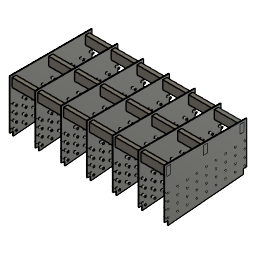
_Shelf Assembly for Animation.40ab5e80-e004-40ce-8bc8-a0c1a8f30ea9 (Autodesk Fusion 360 design; units mm, degrees)
Autodesk Fusion 360 part; units mm, degrees
sketch "Sketch1" plane through (0, 0, 0) normal (0, 0, 1) x (1, 0, 0)
  line L0 (0, 0) -> (6.35, 0)
  line L1 (6.35, 0) -> (6.35, 958.998)
  line L2 (6.35, 1060.598) -> (0, 1060.598)
  line L3 (0, 1060.598) -> (0, 0)
  line L4 (292.7, 0) -> (292.7, 958.998)
  line L5 (286.35, 0) -> (292.7, 0)
  line L6 (286.35, 958.998) -> (286.35, 0)
  line L7 (292.7, 1060.598) -> (286.35, 1060.598)
  line L8 (579.05, 0) -> (579.05, 958.998)
  line L9 (572.7, 0) -> (579.05, 0)
  line L10 (572.7, 958.998) -> (572.7, 0)
  line L11 (579.05, 1060.598) -> (572.7, 1060.598)
  line L12 (865.4, 0) -> (865.4, 958.998)
  line L13 (859.05, 0) -> (865.4, 0)
  line L14 (859.05, 958.998) -> (859.05, 0)
  line L15 (865.4, 1060.598) -> (859.05, 1060.598)
  line L16 (1151.75, 0) -> (1151.75, 958.998)
  line L17 (1145.4, 0) -> (1151.75, 0)
  line L18 (1145.4, 958.998) -> (1145.4, 0)
  line L19 (1151.75, 1060.598) -> (1145.4, 1060.598)
  line L20 (1438.1, 0) -> (1438.1, 958.998)
  line L21 (1431.75, 0) -> (1438.1, 0)
  line L22 (1431.75, 958.998) -> (1431.75, 0)
  line L23 (1438.1, 1060.598) -> (1431.75, 1060.598)
  line L24 (1724.45, 0) -> (1724.45, 1060.598)
  line L25 (1718.1, 0) -> (1724.45, 0)
  line L26 (1718.1, 958.998) -> (1718.1, 0)
  line L27 (1724.45, 1060.598) -> (1718.1, 1060.598)
  line L28 (0, 1060.598) -> (1724.45, 1060.598)
  line L29 (1724.45, 1060.598) -> (1724.45, 958.998)
  line L30 (0, 958.998) -> (0, 1060.598)
  line L31 (286.35, 958.998) -> (6.35, 958.998)
  line L32 (572.7, 958.998) -> (292.7, 958.998)
  line L33 (859.05, 958.998) -> (579.05, 958.998)
  line L34 (1145.4, 958.998) -> (865.4, 958.998)
  line L35 (1718.1, 958.998) -> (1438.1, 958.998)
  line L36 (1431.75, 958.998) -> (1151.75, 958.998)
  point P0 (286.35, 0)
  point P1 (572.7, 0)
  point P2 (859.05, 0)
  point P3 (1145.4, 0)
  point P4 (1431.75, 0)
  point P5 (1718.1, 0)
  dimension "d1" = 6.35
  dimension "d2" = 1060.598
  dimension "d7" = 101.6
  constraint horizontal L0
  constraint vertical L1
  constraint horizontal L2
  constraint vertical L3
  constraint coincident L0.start L3.end
  constraint horizontal L28
  constraint vertical L29
  constraint horizontal L35
  constraint vertical L30
  constraint coincident L24 L29.end
  constraint coincident L6.start L35
  constraint coincident L10.start L35
  constraint coincident L14.start L35
  constraint coincident L18.start L35
  constraint coincident L22.start L35
  constraint collinear L31 L35
  constraint collinear L32 L35
  constraint collinear L33 L35
  constraint collinear L34 L35
  constraint collinear L35 L36
  measures "d1" distance of L0.start L0.end
  measures "d2" distance of L0.start L2.end
  measures "d7" distance of L2.end L30.start
sketch "Sketch3" plane through (0, 0, 0) normal (1, 0, 0) x (0, 0, -1)
  circle A0 centre (-408.3427, 236.1947) radius 5.3675
  circle A1 centre (-195.157, 334.846) radius 5.3675
  line L0 (-380.15, 576.0244) -> (-380.15, 480.7744)
  line L1 (-380.15, 480.7744) -> (-424.6, 480.7744)
  circle A2 centre (-301.7498, 325.5203) radius 5.3675
  line L2 (-411.9, 3.3333) -> (426.3, 76.6663)
  line L3 (-424.6, 576.024) -> (-380.15, 576.0244)
  circle A3 centre (-301.7498, 245.5203) radius 5.3675
  line L4 (464.4, 600.8) -> (-450, 600.8)
  circle A4 centre (-435, 328.3) radius 2.25
  circle A5 centre (-195.157, 254.846) radius 5.3675
  line L5 (-424.6, 480.7744) -> (-424.6, 576.024)
  circle A6 centre (-408.3427, 316.1947) radius 5.3675
  circle A7 centre (-435, 248.3) radius 2.25
  circle A8 centre (124.6215, 282.823) radius 5.3675
  circle A9 centre (337.8072, 381.4743) radius 5.3675
  circle A10 centre (-88.5642, 344.1717) radius 5.3675
  line L6 (-450, 50.8) -> (-411.9, 50.8)
  circle A11 centre (18.0287, 353.4973) radius 5.3675
  line L7 (390.4, 576.024) -> (434.85, 576.0244)
  circle A12 centre (-408.3427, 76.1947) radius 5.3675
  circle A13 centre (-435, 88.3) radius 2.25
  line L8 (426.3, 76.6663) -> (426.3, 130.7996)
  circle A14 centre (337.8072, 141.4743) radius 5.3675
  circle A15 centre (18.0287, 193.4973) radius 5.3675
  circle A16 centre (231.2143, 132.1487) radius 5.3675
  circle A17 centre (444.4, 310.8) radius 5.3675
  circle A18 centre (124.6215, 362.823) radius 5.3675
  line L9 (390.4, 480.7744) -> (390.4, 576.024)
  circle A19 centre (18.0287, 273.4973) radius 5.3675
  line L10 (434.85, 480.7744) -> (390.4, 480.7744)
  circle A20 centre (-195.157, 174.846) radius 5.3675
  circle A21 centre (-301.7498, 85.5203) radius 5.3675
  line L11 (27.35, 480.7744) -> (-17.1, 480.7744)
  line L12 (426.3, 130.7996) -> (464.4, 130.7996)
  line L13 (-17.1, 576.024) -> (27.35, 576.0244)
  circle A22 centre (444.4, 150.8) radius 5.3675
  circle A23 centre (-301.7498, 165.5203) radius 5.3675
  line L14 (-411.9, 50.8) -> (-411.9, 3.3333)
  circle A24 centre (444.4, 230.8) radius 5.3675
  circle A25 centre (-408.3427, 156.1947) radius 5.3675
  circle A26 centre (-195.157, 94.846) radius 5.3675
  circle A27 centre (-435, 168.3) radius 2.25
  line L15 (-17.1, 480.7744) -> (-17.1, 576.024)
  line L16 (-450, 600.8) -> (-450, 50.8)
  circle A28 centre (18.0287, 113.4973) radius 5.3675
  circle A29 centre (231.2143, 372.1487) radius 5.3675
  circle A30 centre (-88.5642, 184.1717) radius 5.3675
  circle A31 centre (444.4, 390.8) radius 5.3675
  circle A32 centre (337.8072, 301.4743) radius 5.3675
  circle A33 centre (337.8072, 221.4743) radius 5.3675
  line L17 (464.4, 130.7996) -> (464.4, 600.8)
  circle A34 centre (231.2143, 212.1487) radius 5.3675
  line L18 (434.85, 576.0244) -> (434.85, 480.7744)
  circle A35 centre (-88.5642, 104.1717) radius 5.3675
  circle A36 centre (124.6215, 122.823) radius 5.3675
  circle A37 centre (124.6215, 202.823) radius 5.3675
  line L19 (27.35, 576.0244) -> (27.35, 480.7744)
  circle A38 centre (-88.5642, 264.1717) radius 5.3675
  circle A39 centre (231.2143, 292.1487) radius 5.3675
  point P0 (-100, 0)
extrude "Extrude2" add sketch "Sketch3" along normal blind 6.35 makes body 1
pattern_linear "R-Pattern1" count 7 spacing 286.35 along (1, 0, 0) of bodies 1 makes body 2 at (286.35, 509.8549, -216.3214) makes body 3 at (572.7, 509.8549, -216.3214) makes body 4 at (859.05, 509.8549, -216.3214) makes body 5 at (1145.4, 509.8549, -216.3214) makes body 6 at (1431.75, 509.8549, -216.3214) makes body 7 at (1718.1, 509.8549, -216.3214)
sketch "Sketch4" plane through (0, 0, 0) normal (-1, 0, 0) x (0, 0, 1)
  circle A0 centre (-124.6215, 202.823) radius 5.3675
  circle A1 centre (408.3427, 156.1947) radius 5.3675
  circle A2 centre (-444.4, 310.8) radius 5.3675
  circle A3 centre (-337.8072, 221.4743) radius 5.3675
  circle A4 centre (-231.2143, 132.1487) radius 5.3675
  circle A5 centre (435, 168.3) radius 2.25
  circle A6 centre (-231.2143, 292.1487) radius 5.3675
  circle A7 centre (-124.6215, 122.823) radius 5.3675
  circle A8 centre (-444.4, 150.8) radius 5.3675
  line L0 (-434.85, 576.0244) -> (-390.4, 576.024)
  line L1 (-390.4, 576.024) -> (-390.4, 480.7744)
  line L2 (-390.4, 480.7744) -> (-434.85, 480.7744)
  line L3 (-434.85, 480.7744) -> (-434.85, 576.0244)
  circle A9 centre (-337.8072, 301.4743) radius 5.3675
  circle A10 centre (195.157, 94.846) radius 5.3675
  circle A11 centre (301.7498, 245.5203) radius 5.3675
  circle A12 centre (301.7498, 85.5203) radius 5.3675
  circle A13 centre (-18.0287, 113.4973) radius 5.3675
  circle A14 centre (301.7498, 165.5203) radius 5.3675
  circle A15 centre (-444.4, 230.8) radius 5.3675
  circle A16 centre (88.5642, 104.1717) radius 5.3675
  circle A17 centre (-231.2143, 212.1487) radius 5.3675
  circle A18 centre (88.5642, 184.1717) radius 5.3675
  circle A19 centre (88.5642, 264.1717) radius 5.3675
  circle A20 centre (-337.8072, 141.4743) radius 5.3675
  circle A21 centre (-231.2143, 372.1487) radius 5.3675
  line L4 (424.6, 480.7744) -> (380.15, 480.7744)
  line L5 (380.15, 480.7744) -> (380.15, 576.0244)
  line L6 (380.15, 576.0244) -> (424.6, 576.024)
  line L7 (424.6, 576.024) -> (424.6, 480.7744)
  circle A22 centre (-124.6215, 362.823) radius 5.3675
  circle A23 centre (195.157, 334.846) radius 5.3675
  circle A24 centre (435, 88.3) radius 2.25
  circle A25 centre (408.3427, 236.1947) radius 5.3675
  circle A26 centre (435, 328.3) radius 2.25
  circle A27 centre (195.157, 254.846) radius 5.3675
  circle A28 centre (195.157, 174.846) radius 5.3675
  circle A29 centre (-444.4, 390.8) radius 5.3675
  circle A30 centre (-18.0287, 193.4973) radius 5.3675
  line L8 (-27.35, 576.0244) -> (17.1, 576.024)
  line L9 (17.1, 576.024) -> (17.1, 480.7744)
  line L10 (17.1, 480.7744) -> (-27.35, 480.7744)
  line L11 (-27.35, 480.7744) -> (-27.35, 576.0244)
  circle A31 centre (-18.0287, 273.4973) radius 5.3675
  circle A32 centre (408.3427, 76.1947) radius 5.3675
  circle A33 centre (435, 248.3) radius 2.25
  circle A34 centre (-337.8072, 381.4743) radius 5.3675
  circle A35 centre (-124.6215, 282.823) radius 5.3675
  circle A36 centre (301.7498, 325.5203) radius 5.3675
  circle A37 centre (88.5642, 344.1717) radius 5.3675
  circle A38 centre (-18.0287, 353.4973) radius 5.3675
  circle A39 centre (408.3427, 316.1947) radius 5.3675
  line L12 (-464.4, 600.8) -> (-464.4, 130.7996)
  line L13 (-464.4, 130.7996) -> (-426.3, 130.7996)
  line L14 (-426.3, 130.7996) -> (-426.3, 76.6663)
  line L15 (-426.3, 76.6663) -> (411.9, 3.3333)
  line L16 (411.9, 3.3333) -> (411.9, 50.8)
  line L17 (411.9, 50.8) -> (450, 50.8)
  line L18 (450, 50.8) -> (450, 600.8)
  line L19 (450, 600.8) -> (-464.4, 600.8)
extrude "Extrude3" add sketch "Sketch4" against normal up to surface (1724.45 mm away) contours L0 L1 L2 L3 | L4 L5 L6 L7 | L8 L9 L10 L11 bodies 1 2 3 4 5 6 7
sketch "Sketch5" plane through (0, 0, 0) normal (-1, 0, 0) x (0, 0, 1)
  circle A0 centre (-124.6215, 202.823) radius 5.3675
  circle A1 centre (408.3427, 156.1947) radius 5.3675
  circle A2 centre (-444.4, 310.8) radius 5.3675
  circle A3 centre (-337.8072, 221.4743) radius 5.3675
  circle A4 centre (-231.2143, 132.1487) radius 5.3675
  circle A5 centre (435, 168.3) radius 2.25
  circle A6 centre (-231.2143, 292.1487) radius 5.3675
  circle A7 centre (-124.6215, 122.823) radius 5.3675
  circle A8 centre (-444.4, 150.8) radius 5.3675
  circle A9 centre (-337.8072, 301.4743) radius 5.3675
  circle A10 centre (195.157, 94.846) radius 5.3675
  circle A11 centre (301.7498, 245.5203) radius 5.3675
  circle A12 centre (301.7498, 85.5203) radius 5.3675
  circle A13 centre (-18.0287, 113.4973) radius 5.3675
  circle A14 centre (301.7498, 165.5203) radius 5.3675
  circle A15 centre (-444.4, 230.8) radius 5.3675
  circle A16 centre (88.5642, 104.1717) radius 5.3675
  circle A17 centre (-231.2143, 212.1487) radius 5.3675
  circle A18 centre (88.5642, 184.1717) radius 5.3675
  circle A19 centre (88.5642, 264.1717) radius 5.3675
  circle A20 centre (-337.8072, 141.4743) radius 5.3675
  circle A21 centre (-231.2143, 372.1487) radius 5.3675
  circle A22 centre (-124.6215, 362.823) radius 5.3675
  circle A23 centre (195.157, 334.846) radius 5.3675
  circle A24 centre (435, 88.3) radius 2.25
  circle A25 centre (408.3427, 236.1947) radius 5.3675
  circle A26 centre (435, 328.3) radius 2.25
  circle A27 centre (195.157, 254.846) radius 5.3675
  circle A28 centre (195.157, 174.846) radius 5.3675
  circle A29 centre (-444.4, 390.8) radius 5.3675
  circle A30 centre (-18.0287, 193.4973) radius 5.3675
  circle A31 centre (-18.0287, 273.4973) radius 5.3675
  circle A32 centre (408.3427, 76.1947) radius 5.3675
  circle A33 centre (435, 248.3) radius 2.25
  circle A34 centre (-337.8072, 381.4743) radius 5.3675
  circle A35 centre (-124.6215, 282.823) radius 5.3675
  circle A36 centre (301.7498, 325.5203) radius 5.3675
  circle A37 centre (88.5642, 344.1717) radius 5.3675
  circle A38 centre (-18.0287, 353.4973) radius 5.3675
  circle A39 centre (408.3427, 316.1947) radius 5.3675
  line L0 (-464.4, 600.8) -> (-464.4, 130.7996)
  line L1 (-464.4, 130.7996) -> (-426.3, 130.7996)
  line L2 (-426.3, 130.7996) -> (-426.3, 76.6663)
  line L3 (-426.3, 76.6663) -> (411.9, 3.3333)
  line L4 (411.9, 3.3333) -> (411.9, 50.8)
  line L5 (411.9, 50.8) -> (450, 50.8)
  line L6 (450, 50.8) -> (450, 600.8)
  line L7 (450, 600.8) -> (-464.4, 600.8)
  circle A40 centre (-444.4, 390.8) radius 11
  dimension "d24" = 22
  constraint concentric A29 A40
  measures "d24" diameter of A40
extrude "Extrude4" add sketch "Sketch5" against normal up to surface (1724.45 mm away) contours A29 | A40 bodies 1
pattern_linear "R-Pattern2" count 4 spacing 80 along (0, -1, 0) count 9 spacing 107 along (0, -0.087156, 0.996195) of "Extrude4"
sketch "Sketch6" plane through (0, 0, -434.85) normal (0, 0, -1) x (-1, 0, 0)
  line L0 (-1438.1, 480.7744) -> (-1438.1, 576.0244)
  line L1 (-1438.1, 576.0244) -> (-1718.1, 576.0244)
  line L2 (-1718.1, 576.0244) -> (-1718.1, 480.7744)
  line L3 (-1718.1, 480.7744) -> (-1438.1, 480.7744)
sketch "Sketch7" plane through (0, 0, -464.4) normal (0, 0, -1) x (-1, 0, 0)
  line L0 (-1718.1, 130.7996) -> (-1718.1, 600.8)
  line L1 (-1718.1, 600.8) -> (-1724.45, 600.8)
  line L2 (-1724.45, 600.8) -> (-1724.45, 130.7996)
  line L3 (-1724.45, 130.7996) -> (-1718.1, 130.7996)
  line L4 (-1685.7, 429.3333) -> (-1470.5, 429.3333)
  line L5 (-1470.5, 429.3333) -> (-1470.5, 5.2956)
  line L6 (-1470.5, 5.2956) -> (-1685.7, 5.2956)
  line L7 (-1685.7, 5.2956) -> (-1685.7, 429.3333)
  dimension "d25" = 215.2
  dimension "d26" = 32.4
  constraint horizontal L4
  constraint vertical L5
  constraint horizontal L6
  constraint vertical L7
  measures "d25" distance of L4.start L4.end
  measures "d26" distance of L0 L7
extrude "Extrude5" cut sketch "Sketch7" against normal blind 1100 contours L4 L5 L6 L7 bodies 1
pattern_linear "R-Pattern3" count 6 spacing 286.35 along (-1, 0, 0) of "Extrude5"
